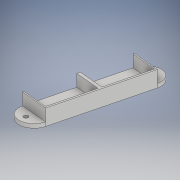
# Autodesk Inventor part: Wago Terminal Block New
Saved by Autodesk Inventor 2018.3 (Build 223285000, 285)
## iProperties
Created: 2021-05-25
Part Number: Wago Terminal Block New
Material: Generic
Document SubType Name: Modeling
Designer: Eugene
Density: 1 g/cm^3
Appearance: Default
Author: Eugene
Autodesk Inventor part; units mm, degrees
ref_plane "YZ Plane" through (0, 0, 0) normal (1, 0, 0) x (0, 1, 0)
ref_plane "XZ Plane" through (0, 0, 0) normal (0, 1, 0) x (-1, 0, 0)
ref_plane "XY Plane" through (0, 0, 0) normal (0, 0, 1) x (1, 0, 0)
sketch "Sketch4" plane through (0, 0, 0) normal (0, 1, 0) x (-1, 0, 0)
  line L0 (0, 0) -> (22.5, 0)
  line L1 (22.5, 0) -> (22.5, -77.5)
  line L2 (22.5, -77.5) -> (0, -77.5)
  line L3 (0, -77.5) -> (0, 0)
  arc A0 (0, -77.5) -> (22.5, -77.5) centre (11.25, -77.5) ccw
  arc A1 (22.5, 0) -> (0, 0) centre (11.25, 0) ccw
  dimension "d13" = 22.5
  dimension "d14" = 77.5
  constraints: 8 end point, 4 point on circle, 4 tangent, 2 centre point, 2 parallel, 1 horizontal, 1 perpendicular
  measures "d13" distance of L1.end L2.end
  measures "d14" distance of L0.end L1.end
extrude "Extrusion10" add sketch "Sketch4" along normal blind 3 contours A1 L0 | L2 A0
sketch "Sketch13" plane through (0, 0, 0) normal (0, -1, 0) x (1, 0, 0)
  line L0 (0, 0) -> (-22.5, 0) projected
  line L1 (-22.5, -77.5) -> (0, -77.5) projected
  line L2 (0, 0) -> (-22.5, 0)
  line L3 (-22.5, 0) -> (-22.5, -77.5)
  line L4 (-22.5, -77.5) -> (0, -77.5)
  line L5 (0, -77.5) -> (0, 0)
  constraints: 8 end point, 2 parallel, 1 horizontal, 1 perpendicular
extrude "Extrusion11" add sketch "Sketch13" against normal blind 3
sketch "Sketch17" plane through (0, 3, 0) normal (0, 1, 0) x (1, 0, 0)
  line L0 (-22.5, 77.5) -> (-22.5, 0) projected
  line L1 (-22.5, 0) -> (-21, 0)
  line L2 (-21, 0) -> (-21, 77.5)
  line L3 (-21, 77.5) -> (-22.5, 77.5)
  line L4 (-22.5, 77.5) -> (-22.5, 0)
  point P0 (0, 0)
  dimension "d82" = 1.5
  constraints: 8 end point, 2 parallel, 1 horizontal, 1 perpendicular
  measures "d82" distance of L3.end L2.end
extrude "Extrusion14" add sketch "Sketch17" along normal blind 9
sketch "Sketch18" plane through (0, 3, 0) normal (0, 1, 0) x (1, 0, 0)
  line L0 (0, 0) -> (0, 77.5) projected
  line L1 (-21, 0) -> (-21, 77.5) projected
  line L2 (0, 0) -> (-21, 0)
  line L3 (-21, 0) -> (-21, 1)
  line L4 (-21, 1) -> (0, 1)
  line L5 (0, 1) -> (0, 0)
  arc A0 (0, 77.5) -> (-22.5, 77.5) centre (-11.25, 77.5) ccw projected
  line L6 (0, 77.5) -> (-21, 77.5)
  line L7 (-21, 77.5) -> (-21, 76.5)
  line L8 (-21, 76.5) -> (0, 76.5)
  line L9 (0, 76.5) -> (0, 77.5)
  line L10 (-21, 37.5) -> (0, 37.5)
  line L11 (0, 37.5) -> (0, 40)
  line L12 (0, 40) -> (-21, 40)
  line L13 (-21, 40) -> (-21, 37.5)
  dimension "d85" = 1
  dimension "d86" = 1
  dimension "d87" = 2.5
  dimension "d88" = 36.5
  constraints: 24 end point, 6 parallel, 4 point on line, 3 horizontal, 3 perpendicular
  measures "d85" distance of L2.end L3.end
  measures "d86" distance of L7.end L6.end
  measures "d87" distance of L11.end L10.end
  measures "d88" distance between parallel lines of L8 L12
extrude "Extrusion15" add sketch "Sketch18" along normal blind 9 contours L2 L1 L4 L0 | L10 L1 L12 L0 | L8 L1 L6 L0
sketch "Sketch19" plane through (0, 3, 0) normal (0, 1, 0) x (1, 0, 0)
  line L0 (0, 77.5) -> (-22.5, 77.5) projected
  circle A0 centre (-11.25, 83.125) radius 1.75
  arc A1 (-22.5, 0) -> (0, 0) centre (-11.25, 0) ccw projected
  circle A2 centre (-11.25, -5.625) radius 1.75
  dimension "d92" = 3.5
  dimension "d94" = 3.5
  constraints: 2 centre point
  measures "d92" diameter of A0
  measures "d94" diameter of A2
hole "Hole3" at (-11.25, 3, -83.125) at (-11.25, 3, 5.625) direction (0, -1, 0) diameter 3.5 end through all
body "Solid4"
